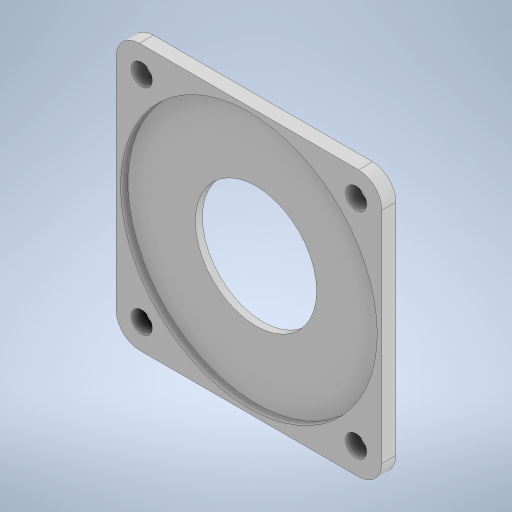
# Autodesk Inventor part: BackPlate
Saved by Autodesk Inventor 2024 (Build 280153000, 153)
## iProperties
Created: 2024-01-27
Part Number: BackPlate
Material: Generic
Document SubType Name: Modeling
Designer: Owner
Density: 1 g/cm^3
Appearance: Default
Author: Owner
Autodesk Inventor part; units mm, degrees
ref_plane "YZ Plane" through (0, 0, 0) normal (1, 0, 0) x (0, 1, 0)
ref_plane "XZ Plane" through (0, 0, 0) normal (0, 1, 0) x (-1, 0, 0)
ref_plane "XY Plane" through (0, 0, 0) normal (0, 0, 1) x (1, 0, 0)
sketch "Sketch1" plane through (0, 0, 0) normal (0, 0, 1) x (1, 0, 0)
  line L0 (0, 0) -> (114, 0)
  line L1 (114, 0) -> (114, 114)
  line L2 (114, 114) -> (0, 114)
  line L3 (0, 114) -> (0, 0)
  dimension "d0" = 114
  dimension "d1" = 114
  constraints: 8 end point, 2 parallel, 1 horizontal, 1 perpendicular
  measures "d0" distance of L1.end L2.end
  measures "d1" distance of L0.end L1.end
extrude "Extrusion1" add sketch "Sketch1" along normal blind 6
sketch "Sketch2" plane through (0, 0, 6) normal (0, 0, 1) x (1, 0, 0)
  circle A0 centre (57, 57) radius 55
  line L0 (0, 114) -> (0, 0) projected
  line L1 (0, 0) -> (114, 0) projected
  dimension "d4" = 110
  dimension "d5" = 57
  dimension "d6" = 57
  constraints: 1 centre point
  measures "d4" diameter of A0
  measures "d5" distance from line of L0 A0.centre
  measures "d6" distance from line of L1 A0.centre
extrude "Extrusion2" cut sketch "Sketch2" against normal blind 3
fillet "Fillet1" radius 10 1 edges at (0, 114, 3)
fillet "Fillet2" radius 10 3 edges at (114, 114, 3) (114, 0, 3) (0, 0, 3)
sketch "Sketch3" plane through (0, 0, 6) normal (0, 0, 1) x (1, 0, 0)
  circle A0 centre (11.038, 11.038) radius 4.5
  line L0 (10, 0) -> (104, 0) projected
  line L1 (0, 104) -> (0, 10) projected
  circle A1 centre (11.038, 102.962) radius 4.5
  circle A2 centre (102.962, 102.962) radius 4.5
  circle A3 centre (102.962, 11.038) radius 4.5
  line L2 (104, 114) -> (10, 114) projected
  line L3 (114, 10) -> (114, 104) projected
  point P0 (0, 0)
  dimension "d11" = 9
  dimension "d12" = 11.038
  dimension "d13" = 11.038
  dimension "d14" = 9
  dimension "d15" = 9
  dimension "d16" = 9
  dimension "d17" = 11.038
  dimension "d18" = 11.038
  dimension "d19" = 11.038
  dimension "d20" = 11.038
  dimension "d21" = 11.038
  dimension "d22" = 11.038
  constraints: 4 centre point
  measures "d11" diameter of A0
  measures "d12" distance from line of L0 A0.centre
  measures "d13" distance from line of L1 A0.centre
  measures "d14" diameter of A1
  measures "d15" diameter of A2
  measures "d16" diameter of A3
  measures "d17" distance from line of L2 A1.centre
  measures "d18" distance from line of L1 A1.centre
  measures "d19" distance from line of L3 A2.centre
  measures "d20" distance from line of L2 A2.centre
  measures "d21" distance from line of L3 A3.centre
  measures "d22" distance from line of L0 A3.centre
extrude "Extrusion3" cut sketch "Sketch3" against normal blind 6
sketch "Sketch4" plane through (57, 57, 3) normal (0, 0, 1) x (1, 0, 0)
  circle A0 centre (0, 0) radius 26
  line L0 (-57, 47) -> (-57, -47) projected
  line L1 (-47, -57) -> (47, -57) projected
  point P0 (-57, -57)
  point P1 (0, -57)
  dimension "d25" = 52
  dimension "d26" = 57
  dimension "d27" = 57
  constraints: 1 centre point, 1 midpoint
  measures "d25" diameter of A0
  measures "d26" distance from line of L0 A0.centre
  measures "d27" distance of A0.centre point (0, -57)
extrude "Extrusion4" cut sketch "Sketch4" against normal blind 10
equation "\"d6\" = d5"
equation "\"d13\" = d12"
equation "\"d17\" = d12"
equation "\"d18\" = d13"
equation "\"d19\" = d18"
equation "\"d20\" = d18"
equation "\"d21\" = d19"
equation "\"d22\" = d21"
body "Solid1"
